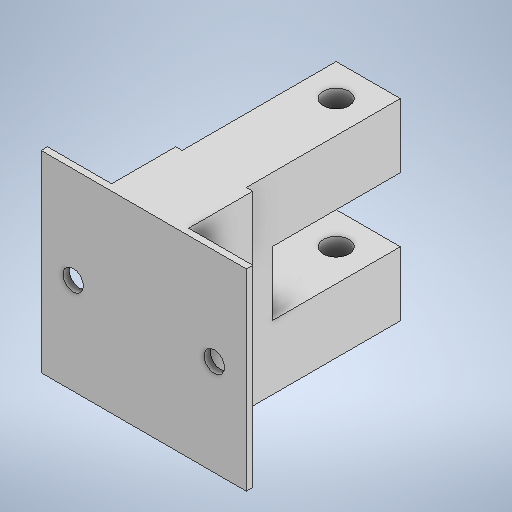
# Autodesk Inventor part: y_bearing_holder
Saved by Autodesk Inventor 2025 (Build 290162000, 162)
## iProperties
Created: 2024-04-25
Part Number: y_bearing_holder
Material: Všeobecné
Document SubType Name: Modeling
Designer: rader
Density: 1 g/cm^3
Appearance: Výchozí
Author: rader
Autodesk Inventor part; units mm, degrees
ref_plane "YZ Plane" through (0, 0, 0) normal (1, 0, 0) x (0, 1, 0)
ref_plane "XZ Plane" through (0, 0, 0) normal (0, 1, 0) x (-1, 0, 0)
ref_plane "XY Plane" through (0, 0, 0) normal (0, 0, 1) x (1, 0, 0)
sketch "Náčrt1" plane through (0, 0, 0) normal (0, 0, 1) x (1, 0, 0)
  line L0 (-9.2032, 0) -> (20.2005, 0) projected
  line L1 (0, 42) -> (0, -7) projected
  line L2 (-5.0026, 0) -> (16, 0)
  line L3 (16, 0) -> (16, 1)
  line L4 (16, 1) -> (6, 1)
  line L5 (6, 1) -> (6, 11)
  line L6 (6, 11) -> (5, 11)
  line L7 (5, 11) -> (5, 35)
  line L8 (5, 35) -> (0, 35)
  line L9 (0, 35) -> (0, 0)
  line L10 (0, 0) -> (-5.0026, 0)
  line L11 (0, 0) -> (16, 0)
  point P0 (0, 0)
  point P1 (0, 35)
  point P2 (16, 0)
  dimension "d0" = 10
  dimension "d1" = 10
  dimension "d2" = 1
  dimension "d3" = 1
  dimension "d4" = 5
  dimension "d5" = 35
  constraints: 20 end point, 7 perpendicular, 3 collinear, 1 horizontal, 1 parallel, 1 point on line
  measures "d0" distance of L3.end L4.end
  measures "d1" distance of L4.end L5.end
  measures "d2" distance between parallel lines of L4 L2
  measures "d3" distance between parallel lines of L7 L5
  measures "d4" distance of L7.end L8.end
  measures "d5" distance of L8.end L9.end
extrude "Vysunutí1" add sketch "Náčrt1" along normal mid plane 30
mirror "Zrcadlit1" about plane through (0, 35, 0) normal (-1, 0, 0) of "Vysunutí1"
sketch "Náčrt2" plane through (5, 11, 15) normal (1, 0, 0) x (0, 0, -1)
  line L0 (0, 24) -> (30, 24) projected
  line L1 (0, 0) -> (0, 24) projected
  line L2 (30, 0) -> (0, 0) projected
  line L3 (30, 24) -> (30, 0) projected
  line L4 (10, 24) -> (20, 24)
  line L5 (20, 24) -> (20, 4)
  line L6 (20, 4) -> (10, 4)
  line L7 (10, 4) -> (10, 24)
  line L8 (10, 24) -> (20, 24)
  point P0 (15, -11)
  point P1 (10, 0)
  point P2 (20, 0)
  dimension "d8" = 10
  dimension "d9" = 10
  dimension "d10" = 20
  constraints: 10 end point, 2 parallel, 2 perpendicular, 1 horizontal, 1 point on line
  measures "d8" distance between parallel lines of L1 L7
  measures "d9" distance of L5.end L6.end
  measures "d10" distance of L4.end L5.end
extrude "Vysunutí3" cut sketch "Náčrt2" against normal through all contours L0 L5 L6 L7
sketch "Náčrt3" plane through (0, 0, 15) normal (0, 0, 1) x (1, 0, 0)
  line L0 (5, 35) -> (-5, 35) projected
  line L1 (-5, 11) -> (-5, 35) projected
  line L2 (-6, 11) -> (-5, 11) projected
  line L3 (-6, 1) -> (-6, 11) projected
  line L4 (-16, 1) -> (-6, 1) projected
  line L5 (-16, 0) -> (-16, 1) projected
  line L6 (16, 0) -> (-16, 0) projected
  line L7 (16, 0) -> (16, 1) projected
  line L8 (16, 1) -> (6, 1) projected
  line L9 (6, 1) -> (6, 11) projected
  line L10 (6, 11) -> (5, 11) projected
  line L11 (5, 11) -> (5, 35) projected
  point P0 (0, 0)
  point P1 (0, 30)
  dimension "d15" = 5
  dimension "d16" = 5
  measures "d15" distance from line of L0 point (0, 30)
  measures "d16" distance from line of L11 point (0, 30)
hole "Díra1" at (0, 30, 15) direction (0, 0, -1) diameter 4 end through all
sketch "Náčrt4" plane through (16, 0, -15) normal (0, -1, 0) x (1, 0, 0)
  line L0 (-10, 0) -> (-10, 30) projected
  line L1 (0, 0) -> (0, 30) projected
  line L2 (0, 30) -> (-32, 30) projected
  line L3 (-32, 0) -> (-32, 30) projected
  line L4 (0, 0) -> (-32, 0) projected
  point P0 (-16, 15)
  point P1 (-5, 15)
  point P2 (-27, 15)
  dimension "d24" = 5
  dimension "d27" = 15
  dimension "d28" = 15
  dimension "d31" = 5
  measures "d24" distance from line of L1 point (-5, 15)
  measures "d27" distance from line of L4 point (-5, 15)
  measures "d28" distance from line of L4 point (-27, 15)
  measures "d31" distance from line of L3 point (-27, 15)
hole "Díra2" at (11, 0, 0) at (-11, 0, 0) direction (0, 1, 0) diameter 3.2 end through all
